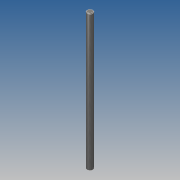
# Autodesk Inventor part: 200-60-DIFFERENTIAL-BAR-05
Saved by Autodesk Inventor 2018.2 (Build 222227000, 227)
## iProperties
Manager: feesmrt
Company: FRANCOR
Part Number: 200-60-DIFFERENTIAL-BAR-05
Project: Rescue Robot
Cost Center: -
Material: Edelstahl
Document SubType Name: Modeling
Designer: feesmrt
Engineer: feesmrt
Authority: feesmrt
Density: 8 g/cm^3
Appearance: Halbpoliert
Description: Gewindestange M8
Stock Number: 200-60-DIFFERENTIAL-BAR-05
Subject: Rescue Robot
Author: feesmrt
Revision Number: 1
Title: Gewindestange M8
Autodesk Inventor part; units mm, degrees
ref_plane "YZ Plane" through (0, 0, 0) normal (1, 0, 0) x (0, 1, 0)
ref_plane "XZ Plane" through (0, 0, 0) normal (0, 1, 0) x (-1, 0, 0)
ref_plane "XY Plane" through (0, 0, 0) normal (0, 0, 1) x (1, 0, 0)
sketch "Skizze3" plane through (0, 0, 0) normal (0, 0, 1) x (1, 0, 0)
  circle A0 centre (0, 0) radius 4
  dimension "d15" = 8
  constraints: 1 centre point, 1 coincident
  measures "d15" diameter of A0
extrude "Grundkörper" add sketch "Skizze3" along normal mid plane 190
thread "M8" size "M8x1.25" class "6g" standard "ANSI Metric M Profile" full length
chamfer "Fase" distance 0.75 angle 45 2 edges at (-4, 0, 95) (-4, 0, -95)
